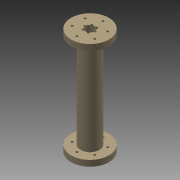
# Autodesk Inventor part: 主动轮连接筒
Saved by Autodesk Inventor 2015 (Build 190159000, 159)
## iProperties
Created: 2017-05-09
Part Number: 主动轮连接筒
Material: 常规
Document SubType Name: Modeling
Designer: Administrator
Density: 1 g/cm^3
Appearance: 麦色
Author: Administrator
Autodesk Inventor part; units mm, degrees
ref_plane "YZ Plane" through (0, 0, 0) normal (1, 0, 0) x (0, 1, 0)
ref_plane "XZ Plane" through (0, 0, 0) normal (0, 1, 0) x (-1, 0, 0)
ref_plane "XY Plane" through (0, 0, 0) normal (0, 0, 1) x (1, 0, 0)
sketch "草图1" plane through (0, 0, 0) normal (0, 0, 1) x (1, 0, 0)
  circle A0 centre (0, 0) radius 80
  dimension "d0" = 160
  constraints: 1 centre point, 1 coincident
  measures "d0" diameter of A0
extrude "拉伸1" add sketch "草图1" along normal blind 25
sketch "草图2" plane through (0, 0, 25) normal (0, 0, 1) x (1, 0, 0)
  circle A0 centre (0, 0) radius 40
  dimension "d3" = 80
  constraints: 1 centre point, 1 coincident
  measures "d3" diameter of A0
extrude "拉伸2" add sketch "草图2" along normal blind 400
sketch "草图3" plane through (0, 0, 0) normal (0, 0, -1) x (-1, 0, 0)
  circle A0 centre (0, 55) radius 4.7538
  line L0 (0, 0) -> (0, 9.1463)
  dimension "d6" = 9.1463
  dimension "d7" = 55
  constraints: 2 end point, 1 centre point, 1 point on line, 1 vertical
  measures "d6" distance of L0.start L0.end
  measures "d7" distance of L0.start A0.centre
extrude "拉伸3" cut sketch "草图3" against normal through all
pattern_circular "环形阵列1" count 6 over 360 about axis through (0, 0, -10) along (0, 0, 1) of "拉伸3"
pattern_linear "矩形阵列1" count 2 spacing 425 along (0, 0, 1) of "拉伸3", "环形阵列1", "拉伸1"
sketch "草图4" plane through (0, 0, 0) normal (0, 0, -1) x (-1, 0, 0)
  circle A0 centre (0, 0) radius 20
  dimension "d16" = 40
  constraints: 1 centre point, 1 coincident
  measures "d16" diameter of A0
extrude "拉伸4" cut sketch "草图4" against normal through all
sketch "草图5" plane through (0, 0, 0) normal (0, 0, -1) x (-1, 0, 0)
  circle A0 centre (0, 0) radius 25
  circle A1 centre (0, 0) radius 20
  circle A2 centre (0, 0) radius 20 projected
  line L0 (24.6779, 4) -> (19.5959, 4)
  line L1 (24.6779, -4) -> (19.5959, -4)
  line L2 (0, 0) -> (7.5201, 0)
  dimension "d19" = 50
  dimension "d20" = 7.5201
  dimension "d21" = 4
  dimension "d22" = 8
  constraints: 6 end point, 6 point on circle, 2 centre point, 2 coincident, 2 parallel, 1 concentric, 1 horizontal
  measures "d19" diameter of A0
  measures "d20" distance of L2.start L2.end
  measures "d21" distance between parallel lines of L2 L0
  measures "d22" distance between parallel lines of L0 L1
extrude "拉伸5" cut sketch "草图5" against normal through all contours A0 L1 A1 L0 picked at (21.5439, 2.2304)
pattern_circular "环形阵列2" count 6 over 360 about axis through (0, 0, -10) along (0, 0, 1) of "拉伸5"
